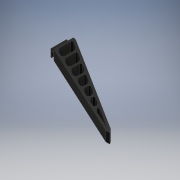
# Autodesk Inventor part: leg
Saved by Autodesk Inventor 2017 (Build 210142000, 142)
## iProperties
Created: 2020-06-17
Part Number: leg
Material: ABS Plastic
Document SubType Name: Modeling
Designer: HAYNIE R&D
Density: 1.06 g/cm^3
Appearance: Glossy - Black
Mass: 111.111 g
Surface Area: 435.041 cm^2
Volume: 104.822 cm^3
Author: HAYNIE R&D
Autodesk Inventor part; units mm, degrees
ref_plane "YZ Plane" through (0, 0, 0) normal (1, 0, 0) x (0, 1, 0)
ref_plane "XZ Plane" through (0, 0, 0) normal (0, 1, 0) x (-1, 0, 0)
ref_plane "XY Plane" through (0, 0, 0) normal (0, 0, 1) x (1, 0, 0)
sketch "Sketch1" plane through (0, 0, 0) normal (0, 0, 1) x (1, 0, 0)
  line L0 (0, 113.4196) -> (0, 163.4196)
  line L1 (0, 163.4196) -> (5, 163.4196)
  line L2 (5, 163.4196) -> (256, 5.04)
  line L3 (256, 5.04) -> (256, 0.0001)
  line L4 (256, 0.0001) -> (246, 0.0001)
  line L5 (256, 0.0001) -> (266, 0.0001) construction
  line L6 (246, 0.0001) -> (0, 113.4196)
  dimension "d1" = 50
  dimension "d2" = 163.4196
  dimension "d5" = 5
  dimension "d14" = 10
  dimension "d15" = 180
  constraints: 14 end point, 3 horizontal, 2 vertical, 1 collinear
  measures "d1" distance of L0.start L0.end
  measures "d2" vertical distance of L3.end L0.end
  measures "d5" distance of L0.end L1.end
  measures "d14" distance of L3.end L4.end
  measures "d15" angle of L4 L5
extrude "Extrusion1" add sketch "Sketch1" along normal blind 25
shell "Shell3" thickness 5 removed faces 2 at (83.6667, 92.2798, 25) at (83.6667, 92.2798, 0)
sketch "Sketch4" plane through (0, 0, 25) normal (0, 0, 1) x (1, 0, 0)
  line L0 (30, 141.7326) -> (30, 105.0938)
  line L1 (245.599, 5.6908) -> (5, 116.6202) projected
  line L2 (35, 102.7885) -> (35, 138.5776)
  line L3 (5, 157.5075) -> (245.599, 5.6908) projected
  line L4 (30, 105.0938) -> (35, 102.7885)
  line L5 (30, 141.7326) -> (35, 138.5776)
  line L6 (5, 116.6202) -> (5, 157.5075) projected
  line L7 (60, 122.8028) -> (60, 91.2622)
  line L8 (65, 119.6478) -> (65, 88.9569)
  line L9 (60, 122.8028) -> (65, 119.6478)
  line L10 (60, 91.2622) -> (65, 88.9569)
  line L11 (90, 103.8729) -> (90, 77.4305)
  line L12 (95, 100.7179) -> (95, 75.1252)
  line L13 (90, 103.8729) -> (95, 100.7179)
  line L14 (90, 77.4305) -> (95, 75.1252)
  line L15 (120, 84.9431) -> (120, 63.5989)
  line L16 (125, 81.7881) -> (125, 61.2936)
  line L17 (120, 84.9431) -> (125, 81.7881)
  line L18 (120, 63.5989) -> (125, 61.2936)
  line L19 (150, 66.0132) -> (150, 49.7672)
  line L20 (155, 62.8583) -> (155, 47.4619)
  line L21 (149.9292, 66.0579) -> (155, 62.8583)
  line L22 (150, 49.7672) -> (155, 47.4619)
  line L23 (180, 47.0834) -> (180, 35.9355)
  line L24 (185, 43.9284) -> (185, 33.6303)
  line L25 (180, 47.0834) -> (185, 43.9284)
  line L26 (180, 35.9355) -> (185, 33.6303)
  point P0 (0, 0)
  dimension "d22" = 25
  dimension "d23" = 5
  dimension "d26" = 25
  dimension "d28" = 5
  dimension "d31" = 25
  dimension "d32" = 5
  dimension "d33" = 25
  dimension "d34" = 5
  dimension "d35" = 25
  dimension "d36" = 5
  dimension "d37" = 25
  dimension "d38" = 5
  constraints: 48 end point, 10 vertical, 1 point on line, 28 other
  measures "d22" distance between parallel lines of L0 L6
  measures "d23" distance between parallel lines of L2 L0
  measures "d26" distance between parallel lines of L7 L2
  measures "d28" distance between parallel lines of L8 L7
  measures "d31" distance between parallel lines of L11 L8
  measures "d32" distance between parallel lines of L12 L11
  measures "d33" distance between parallel lines of L15 L12
  measures "d34" distance between parallel lines of L16 L15
  measures "d35" distance between parallel lines of L19 L16
  measures "d36" distance between parallel lines of L20 L19
  measures "d37" distance between parallel lines of L23 L20
  measures "d38" distance between parallel lines of L24 L23
extrude "Extrusion4" add sketch "Sketch4" against normal blind 25 contours L3 L2 L1 L0 | L3 L8 L1 L7 | L3 L12 L1 L11 | L3 L16 L1 L15 | L19 L3 L20 L1 | L23 L3 L24 L1
chamfer "Chamfer1" distance 5 angle 45 1 edges at (256, 5.04, 12.5)
fillet "Fillet1" radius 20 1 edges at (5, 163.4196, 12.5)
fillet "Fillet2" radius 20 1 edges at (251.7714, 7.7082, 12.5)
chamfer "Chamfer3" distance 5 angle 45 6 edges at (35, 102.7885, 12.5) (65, 88.9569, 12.5) (95, 75.1252, 12.5) (125, 61.2936, 12.5) (155, 47.4619, 12.5) (185, 33.6303, 12.5)
chamfer "Chamfer4" distance 5 angle 45 7 edges at (30, 105.0938, 12.5) (60, 91.2622, 12.5) (90, 77.4305, 12.5) (120, 63.5989, 12.5) (150, 49.7672, 12.5) (180, 35.9355, 12.5) (245.599, 5.6908, 12.5)
chamfer "Chamfer5" distance 5 angle 45 6 edges at (30, 141.7326, 12.5) (60, 122.8028, 12.5) (90, 103.8729, 12.5) (120, 84.9431, 12.5) (150, 66.0132, 12.5) (180, 47.0834, 12.5)
chamfer "Chamfer6" distance 5 angle 45 7 edges at (5, 157.5075, 12.5) (35, 138.5776, 12.5) (65, 119.6478, 12.5) (95, 100.7179, 12.5) (125, 81.7881, 12.5) (155, 62.8583, 12.5) (185, 43.9284, 12.5)
chamfer "Chamfer7" distance 5 angle 45 1 edges at (5, 116.6202, 12.5)
sketch "Sketch5" plane through (0, 113.4196, 0) normal (-1, 0, 0) x (0, 0, 1)
  line L0 (26.875, 1.25) -> (36.25, 1.25) construction
  line L1 (7.5, -0.0169) -> (17.5, -0.0169)
  line L2 (17.5, -0.0169) -> (17.5, 24.9831)
  line L3 (17.5, 24.9831) -> (7.5, 24.9831)
  line L4 (7.5, 24.9831) -> (7.5, -0.0169)
  line L5 (0, 0) -> (0, 50) projected
  line L6 (25, 50) -> (25, 0) projected
  point P0 (0, -113.4196)
  dimension "d67" = 25
  dimension "d70" = 7.5
  dimension "d71" = 7.5
  dimension "d72" = 10
  constraints: 10 end point, 2 horizontal, 2 parallel, 1 perpendicular
  measures "d67" distance of L2.end L1.end
  measures "d70" distance between parallel lines of L5 L4
  measures "d71" distance between parallel lines of L6 L2
  measures "d72" distance between parallel lines of L2 L4
extrude "Extrusion5" add sketch "Sketch5" along normal blind 5.125
sketch "Sketch7" plane through (-5.125, 113.4196, 0) normal (-1, 0, 0) x (0, 0, 1)
  line L0 (17.5, 0) -> (25, 0) projected
  line L1 (3, 40) -> (22, 40)
  line L2 (22, 40) -> (22, 0)
  line L3 (22, 0) -> (3, 0)
  line L4 (3, 0) -> (3, 40)
  line L5 (25, 50) -> (25, 0) projected
  line L6 (0, 0) -> (0, 50) projected
  point P0 (0, -113.4196)
  dimension "d73" = 3
  dimension "d74" = 3
  dimension "d75" = 19
  dimension "d76" = 40
  constraints: 8 end point, 2 parallel, 1 horizontal, 1 perpendicular, 1 point on line
  measures "d73" distance between parallel lines of L5 L2
  measures "d74" distance between parallel lines of L4 L6
  measures "d75" distance between parallel lines of L2 L4
  measures "d76" distance of L2.end L1.end
extrude "Extrusion6" add sketch "Sketch7" along normal blind 2.5
move or copy body "Move Body1" bodies to move or copy 1 copy no translate (7.75, 0, 0)
sketch "Sketch12" plane through (17.6144, 160.3502, 25) normal (0.5336397, 0.8457119, 0) x (0.8457119, -0.5336397, 0)
  line L0 (-0.1306, 25.3339) -> (282.4201, 25.3339) construction
  line L1 (282.4201, 25.3339) -> (282.4201, 0.3091) construction
  line L2 (282.4201, 0.3091) -> (-0.1306, 0.3091) construction
  line L3 (-0.1306, 0.3091) -> (-0.1306, 25.3339) construction
  line L4 (109.9657, 7.8215) -> (108.6366, 7.8215)
  line L5 (108.6366, 7.8215) -> (108.6366, 12.7161)
  line L6 (108.6366, 12.7161) -> (104.0337, 12.7161)
  line L7 (104.0337, 12.7161) -> (104.0337, 7.8215)
  line L8 (104.0337, 7.8215) -> (102.7047, 7.8215)
  line L9 (102.7047, 7.8215) -> (102.7047, 17.8215)
  line L10 (102.7047, 17.8215) -> (104.0337, 17.8215)
  line L11 (104.0337, 17.8215) -> (104.0337, 13.8993)
  line L12 (104.0337, 13.8993) -> (108.6366, 13.8993)
  line L13 (108.6366, 13.8993) -> (108.6366, 17.8215)
  line L14 (108.6366, 17.8215) -> (109.9657, 17.8215)
  line L15 (109.9657, 17.8215) -> (109.9657, 7.8215)
  line L16 (110.9138, 7.8215) -> (114.2849, 17.8215)
  line L17 (114.2849, 17.8215) -> (115.9219, 17.8215)
  line L18 (115.9219, 17.8215) -> (119.293, 7.8215)
  line L19 (119.293, 7.8215) -> (117.8911, 7.8215)
  line L20 (117.8911, 7.8215) -> (116.9835, 10.6173)
  line L21 (116.9835, 10.6173) -> (113.1666, 10.6173)
  line L22 (113.1666, 10.6173) -> (112.259, 7.8215)
  line L23 (112.259, 7.8215) -> (110.9138, 7.8215)
  line L24 (116.6188, 11.7518) -> (115.071, 16.4601)
  line L25 (115.071, 16.4601) -> (113.5313, 11.7518)
  line L26 (113.5313, 11.7518) -> (116.6188, 11.7518)
  line L27 (127.2428, 17.8215) -> (123.8636, 12.2461)
  line L28 (123.8636, 12.2461) -> (123.8636, 7.8215)
  line L29 (123.8636, 7.8215) -> (122.5345, 7.8215)
  line L30 (122.5345, 7.8215) -> (122.5345, 12.1084)
  line L31 (122.5345, 12.1084) -> (119.1553, 17.8215)
  line L32 (119.1553, 17.8215) -> (120.6302, 17.8215)
  line L33 (120.6302, 17.8215) -> (123.2072, 13.4212)
  line L34 (123.2072, 13.4212) -> (125.8328, 17.8215)
  line L35 (125.8328, 17.8215) -> (127.2428, 17.8215)
  line L36 (135.3222, 7.8215) -> (133.8311, 7.8215)
  line L37 (133.8311, 7.8215) -> (129.4065, 16.4438)
  line L38 (129.4065, 16.4438) -> (129.4065, 7.8215)
  line L39 (129.4065, 7.8215) -> (128.1666, 7.8215)
  line L40 (128.1666, 7.8215) -> (128.1666, 17.8215)
  line L41 (128.1666, 17.8215) -> (130.0548, 17.8215)
  line L42 (130.0548, 17.8215) -> (134.0824, 9.9041)
  line L43 (134.0824, 9.9041) -> (134.0824, 17.8215)
  line L44 (134.0824, 17.8215) -> (135.3222, 17.8215)
  line L45 (135.3222, 17.8215) -> (135.3222, 7.8215)
  line L46 (140.8328, 7.8215) -> (136.9592, 7.8215)
  line L47 (136.9592, 7.8215) -> (136.9592, 8.8425)
  line L48 (136.9592, 8.8425) -> (138.2315, 8.8425)
  line L49 (138.2315, 8.8425) -> (138.2315, 16.8004)
  line L50 (138.2315, 16.8004) -> (136.9592, 16.8004)
  line L51 (136.9592, 16.8004) -> (136.9592, 17.8215)
  line L52 (136.9592, 17.8215) -> (140.8328, 17.8215)
  line L53 (140.8328, 17.8215) -> (140.8328, 16.8004)
  line L54 (140.8328, 16.8004) -> (139.5605, 16.8004)
  line L55 (139.5605, 16.8004) -> (139.5605, 8.8425)
  line L56 (139.5605, 8.8425) -> (140.8328, 8.8425)
  line L57 (140.8328, 8.8425) -> (140.8328, 7.8215)
  line L58 (142.4778, 7.8215) -> (142.4778, 17.8215)
  line L59 (142.4778, 17.8215) -> (148.7339, 17.8215)
  line L60 (148.7339, 17.8215) -> (148.7339, 16.6383)
  line L61 (148.7339, 16.6383) -> (143.8068, 16.6383)
  line L62 (143.8068, 16.6383) -> (143.8068, 13.8993)
  line L63 (143.8068, 13.8993) -> (148.4016, 13.8993)
  line L64 (148.4016, 13.8993) -> (148.4016, 12.7161)
  line L65 (148.4016, 12.7161) -> (143.8068, 12.7161)
  line L66 (143.8068, 12.7161) -> (143.8068, 9.0046)
  line L67 (143.8068, 9.0046) -> (148.7339, 9.0046)
  line L68 (148.7339, 9.0046) -> (148.7339, 7.8215)
  line L69 (148.7339, 7.8215) -> (142.4778, 7.8215)
  line L70 (162.2266, 7.8215) -> (160.5005, 7.8215)
  line L71 (160.5005, 7.8215) -> (157.3401, 11.8004)
  line L72 (157.3401, 11.8004) -> (155.8166, 11.8004)
  line L73 (155.8166, 11.8004) -> (155.8166, 7.8215)
  line L74 (155.8166, 7.8215) -> (154.4875, 7.8215)
  line L75 (154.4875, 7.8215) -> (154.4875, 17.8215)
  line L76 (154.4875, 17.8215) -> (157.0645, 17.8215)
  spline S0 degree 2 poles (157.0645, 17.8215) (157.9235, 17.8215) (159.0824, 17.6351) (159.6091, 17.2947) knots 0 0 0 1 2 2 2
  spline S1 degree 2 poles (159.6091, 17.2947) (160.1358, 16.9544) (160.7436, 15.8928) (160.7436, 15.1067) knots 0 0 0 1 2 2 2
  spline S2 degree 2 poles (160.7436, 15.1067) (160.7436, 14.0127) (159.6253, 12.5297) (158.6691, 12.1732) knots 0 0 0 1 2 2 2
  line L77 (158.6691, 12.1732) -> (162.2266, 7.8215)
  spline S3 degree 2 poles (159.3579, 15.0014) (159.3579, 15.439) (159.0499, 16.1116) (158.7258, 16.3304) knots 0 0 0 1 2 2 2
  spline S4 degree 2 poles (158.7258, 16.3304) (158.4422, 16.5168) (157.6885, 16.6707) (157.1375, 16.6707) knots 0 0 0 1 2 2 2
  line L78 (157.1375, 16.6707) -> (155.8166, 16.6707)
  line L79 (155.8166, 16.6707) -> (155.8166, 12.9106)
  line L80 (155.8166, 12.9106) -> (156.9835, 12.9106)
  spline S5 degree 2 poles (156.9835, 12.9106) (157.5589, 12.9106) (158.4746, 13.1132) (158.7906, 13.4293) knots 0 0 0 1 2 2 2
  spline S6 degree 2 poles (158.7906, 13.4293) (159.0824, 13.7048) (159.3579, 14.4827) (159.3579, 15.0014) knots 0 0 0 1 2 2 2
  line L81 (171.708, 7.8215) -> (169.99, 7.8215)
  line L82 (169.99, 7.8215) -> (168.6204, 9.2558)
  spline S7 degree 2 poles (168.6204, 9.2558) (167.9397, 8.3806) (166.4973, 7.6108) (165.5815, 7.6108) knots 0 0 0 1 2 2 2
  spline S8 degree 2 poles (165.5815, 7.6108) (164.2282, 7.6108) (162.4616, 9.2477) (162.4616, 10.5686) knots 0 0 0 1 2 2 2
  spline S9 degree 2 poles (162.4616, 10.5686) (162.4616, 11.144) (162.7858, 12.0435) (163.0532, 12.4082) knots 0 0 0 1 2 2 2
  spline S10 degree 2 poles (163.0532, 12.4082) (163.3125, 12.7566) (164.0013, 13.2915) (164.3093, 13.486) knots 0 0 0 1 2 2 2
  spline S11 degree 2 poles (164.3093, 13.486) (163.6366, 13.9398) (162.964, 14.9528) (162.964, 15.7145) knots 0 0 0 1 2 2 2
  spline S12 degree 2 poles (162.964, 15.7145) (162.964, 16.1926) (163.3449, 17.003) (163.6529, 17.3109) knots 0 0 0 1 2 2 2
  spline S13 degree 2 poles (163.6529, 17.3109) (163.977, 17.627) (165.0062, 18.0322) (165.614, 18.0322) knots 0 0 0 1 2 2 2
  spline S14 degree 2 poles (165.614, 18.0322) (166.7323, 18.0322) (168.1423, 16.8571) (168.1423, 15.9576) knots 0 0 0 1 2 2 2
  spline S15 degree 2 poles (168.1423, 15.9576) (168.1423, 15.6254) (167.9721, 14.9203) (167.7533, 14.5962) knots 0 0 0 1 2 2 2
  spline S16 degree 2 poles (167.7533, 14.5962) (167.5264, 14.2639) (166.8133, 13.6886) (166.2136, 13.4698) knots 0 0 0 1 2 2 2
  line L83 (166.2136, 13.4698) -> (168.5718, 11.0387)
  spline S17 degree 2 poles (168.5718, 11.0387) (168.661, 11.5897) (168.7015, 12.8863) (168.7015, 13.9317) knots 0 0 0 1 2 2 2
  line L84 (168.7015, 13.9317) -> (170.0143, 13.9317)
  line L85 (170.0143, 13.9317) -> (170.0143, 13.2834)
  spline S18 degree 2 poles (170.0143, 13.2834) (170.0143, 12.6432) (169.6901, 11.0225) (169.3093, 10.2931) knots 0 0 0 1 2 2 2
  line L86 (169.3093, 10.2931) -> (171.708, 7.8215)
  line L87 (168.037, 9.8474) -> (164.9495, 13.0079)
  spline S19 degree 2 poles (164.9495, 13.0079) (164.7874, 12.9025) (164.4551, 12.6027) (164.2525, 12.3109) knots 0 0 0 1 2 2 2
  spline S20 degree 2 poles (164.2525, 12.3109) (164.0905, 12.0759) (163.8473, 11.3142) (163.8473, 10.8928) knots 0 0 0 1 2 2 2
  spline S21 degree 2 poles (163.8473, 10.8928) (163.8473, 9.9366) (164.9819, 8.7048) (165.9462, 8.7048) knots 0 0 0 1 2 2 2
  spline S22 degree 2 poles (165.9462, 8.7048) (166.5864, 8.7048) (167.6156, 9.2477) (168.037, 9.8474) knots 0 0 0 1 2 2 2
  spline S23 degree 2 poles (165.5815, 13.9479) (165.9543, 14.0776) (166.4486, 14.5071) (166.5864, 14.7583) knots 0 0 0 1 2 2 2
  spline S24 degree 2 poles (166.5864, 14.7583) (166.708, 14.9933) (166.8295, 15.52) (166.8295, 15.828) knots 0 0 0 1 2 2 2
  spline S25 degree 2 poles (166.8295, 15.828) (166.8295, 16.4763) (166.0678, 17.1894) (165.5653, 17.1894) knots 0 0 0 1 2 2 2
  spline S26 degree 2 poles (165.5653, 17.1894) (164.9657, 17.1894) (164.2768, 16.379) (164.2768, 15.7793) knots 0 0 0 1 2 2 2
  spline S27 degree 2 poles (164.2768, 15.7793) (164.2768, 15.5119) (164.3741, 15.1229) (164.5362, 14.8717) knots 0 0 0 1 2 2 2
  spline S28 degree 2 poles (164.5362, 14.8717) (164.682, 14.661) (165.1845, 14.191) (165.5815, 13.9479) knots 0 0 0 1 2 2 2
  spline S29 degree 2 poles (180.1683, 12.8134) (180.1683, 11.4438) (179.058, 9.2396) (178.1261, 8.6237) knots 0 0 0 1 2 2 2
  spline S30 degree 2 poles (178.1261, 8.6237) (177.3644, 8.1456) (175.8003, 7.8215) (174.5848, 7.8215) knots 0 0 0 1 2 2 2
  line L88 (174.5848, 7.8215) -> (172.2833, 7.8215)
  line L89 (172.2833, 7.8215) -> (172.2833, 17.8215)
  line L90 (172.2833, 17.8215) -> (174.5605, 17.8215)
  spline S31 degree 2 poles (174.5605, 17.8215) (175.9705, 17.8215) (177.5751, 17.4001) (178.1423, 17.0273) knots 0 0 0 1 2 2 2
  spline S32 degree 2 poles (178.1423, 17.0273) (179.1067, 16.3871) (180.1683, 14.272) (180.1683, 12.8134) knots 0 0 0 1 2 2 2
  spline S33 degree 2 poles (178.7825, 12.8296) (178.7825, 13.9803) (178.0208, 15.6092) (177.2671, 16.0711) knots 0 0 0 1 2 2 2
  spline S34 degree 2 poles (177.2671, 16.0711) (176.7323, 16.3871) (175.5248, 16.6707) (174.6253, 16.6707) knots 0 0 0 1 2 2 2
  line L91 (174.6253, 16.6707) -> (173.6123, 16.6707)
  line L92 (173.6123, 16.6707) -> (173.6123, 8.9722)
  line L93 (173.6123, 8.9722) -> (174.6253, 8.9722)
  spline S35 degree 2 poles (174.6253, 8.9722) (175.5086, 8.9722) (176.8457, 9.2558) (177.3887, 9.6367) knots 0 0 0 1 2 2 2
  spline S36 degree 2 poles (177.3887, 9.6367) (178.0856, 10.1067) (178.7825, 11.6626) (178.7825, 12.8296) knots 0 0 0 1 2 2 2
  point P0 (70.6725, 25)
  constraints: 2 other
extrude "Extrusion8" cut sketch "Sketch12" against normal blind 2
body "Solid1"
